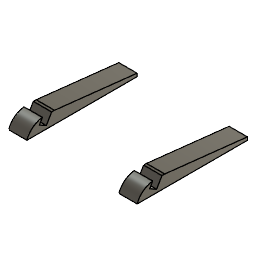
DIY MONITOR STAND (Autodesk Fusion 360 design; units mm, degrees)
part number: 2026-07-20-22-16-48-853
Autodesk Fusion 360 part; units mm, degrees
sketch "Skizze1" plane through (0, 0, 0) normal (0, 0, 1) x (1, 0, 0)
  line L0 (0, 0) -> (350, 0)
  line L1 (350, 0) -> (350, 265)
  line L2 (350, 265) -> (0, 265)
  line L3 (0, 265) -> (0, 0)
  dimension "d1" = 350
  dimension "d2" = 265
  constraint horizontal L0
  constraint vertical L1
  constraint horizontal L2
  constraint vertical L3
  constraint coincident L0.start L3.end
  measures "d1" distance of L0.start L0.end
  measures "d2" distance of L0.start L2.end
extrude "Extrusion1" add sketch "Skizze1" along normal blind 13 makes body 1
move_body "Verschieben1" bodies 1 to x (1, 0, 0) y (0, 0.5, 0.866025) z (0, -0.866025, 0.5) at (0, 121.721, -95.721)
move_body "Verschieben2" bodies 1 to x (1, 0, 0) y (0, 1, 0) z (0, 0, 1) at (0, 0, 110)
sketch "Skizze2" plane through (0, 0, 0) normal (0, 0, 1) x (1, 0, 0)
  line L0 (100, 90) -> (70, 90)
  line L1 (70, 90) -> (70, 190)
  line L2 (100, 190) -> (100, 90)
  line L3 (250, 90) -> (280, 90)
  line L4 (280, 90) -> (280, 190)
  line L5 (280, 190) -> (250, 190)
  line L6 (250, 190) -> (250, 90)
  line L7 (280, 190) -> (280, 270)
  line L8 (280, 270) -> (250, 270)
  line L9 (250, 270) -> (250, 190)
  line L10 (100, 190) -> (70, 190)
  line L11 (70, 190) -> (70, 270)
  line L12 (70, 270) -> (100, 270)
  line L13 (100, 270) -> (100, 190)
  dimension "d8" = 100
  dimension "d9" = 100
  dimension "d22" = 80
  dimension "d23" = 80
  constraint horizontal L0
  constraint vertical L1
  constraint vertical L2
  constraint horizontal L3
  constraint vertical L4
  constraint horizontal L5
  constraint vertical L6
  constraint vertical L7
  constraint horizontal L8
  constraint vertical L9
  constraint horizontal L10
  constraint vertical L11
  constraint horizontal L12
  constraint vertical L13
  measures "d8" distance of L0.start L2.start
  measures "d9" distance of L3.start L5.end
  measures "d22" distance of L5.end L8.end
  measures "d23" distance of L2.start L12.end
extrude "Extrusion2" add sketch "Skizze2" along normal blind 20 separate body makes body 2 at (90, 150, 0) makes body 3 at (270, 150, 0)
move_body "Verschieben3" bodies 1 to x (1, 0, 0) y (0, 1, 0) z (0, 0, 1) at (0, 0, -10)
move_body "Verschieben4" bodies 1 to x (1, 0, 0) y (0, 1, 0) z (0, 0, 1) at (0, 0, 0.721)
fillet "Abrundung1" radius 30 2 edges at (85, 90, 20) (265, 90, 20) on bodies 2 3
chamfer "Fase2" distance 135 distance2 15 2 edges at (265, 270, 20) (85, 270, 20) measured on face at (260, 219.4281, 20) measured on face at (90, 168.8562, 20) on bodies 2 3
combine "Kombinieren1" operation cut target body 3 tool bodies 1 keep tools
combine "Kombinieren2" operation cut target body 2 tool bodies 1 keep tools
hidden bodies 1
